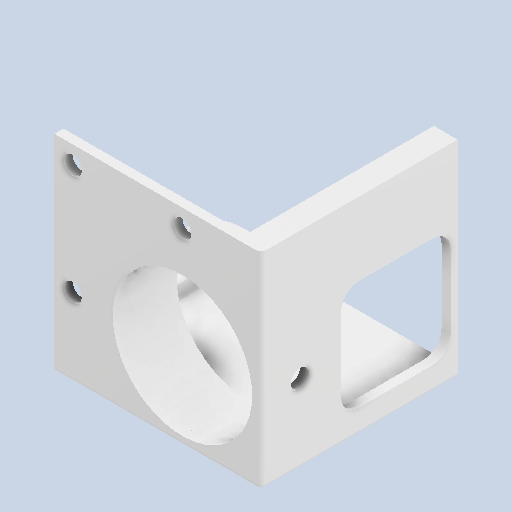
# Autodesk Inventor part: MirrorFix
Saved by Autodesk Inventor 2023 (Build 270158000, 158)
## iProperties
Created: 2022-08-19
Part Number: MirrorFix
Material: ABS Plastic
Document SubType Name: Modeling
Designer: Miner
Density: 1.06 g/cm^3
Appearance: Smooth - White
Author: Miner
Autodesk Inventor part; units mm, degrees
ref_plane "YZ Plane" through (0, 0, 0) normal (1, 0, 0) x (0, 1, 0)
ref_plane "XZ Plane" through (0, 0, 0) normal (0, 1, 0) x (-1, 0, 0)
ref_plane "XY Plane" through (0, 0, 0) normal (0, 0, 1) x (1, 0, 0)
sketch "Sketch1" plane through (0, 0, 0) normal (0, 0, 1) x (1, 0, 0)
  circle A0 centre (0, 0) radius 15 construction
  line L0 (0, 0) -> (0, -12) construction
  line L1 (0, -12) -> (0, 28) construction
  line L2 (0, 28) -> (12, 28) construction
  line L3 (12, 28) -> (-28, 28) construction
  line L4 (-28, 28) -> (-28, -12) construction
  line L5 (-28, -12) -> (12, -12) construction
  line L6 (12, -12) -> (12, 28) construction
  line L7 (-28, 28) -> (17.2, 28)
  line L8 (17.2, 28) -> (17.2, -17.2)
  line L9 (17.2, -17.2) -> (-28, -17.2)
  line L10 (-28, -17.2) -> (-28, 28)
  circle A1 centre (0, 0) radius 15.25
  line L11 (0, -15.25) -> (0, -17.25) construction
  line L12 (-28, -17.2) -> (17.2, -17.2)
  line L13 (17.2, -17.2) -> (17.2, -15.3)
  line L14 (-28, -15.3) -> (-28, -17.2)
  line L15 (17.2, 28) -> (15.3, 28)
  line L16 (17.2, -15.3) -> (17.2, 28)
  circle A2 centre (0, 0) radius 16.85
  line L17 (15.25, 0) -> (17.25, 0) construction
  line L18 (-28, -17.2) -> (17.2, -17.2)
  line L19 (17.2, -17.2) -> (17.2, -15.2)
  line L20 (17.2, -15.2) -> (-28, -15.2)
  line L21 (-28, -15.2) -> (-28, -17.2)
  line L22 (17.2, -15.2) -> (15.2, -15.2)
  line L23 (15.2, -15.2) -> (15.2, 28)
  line L24 (15.2, 28) -> (17.2, 28)
  line L25 (17.2, 28) -> (17.2, -15.2)
  line L26 (-28, -12) -> (-26, -12)
  line L27 (-26, -12) -> (-26, -15.2)
  line L28 (-26, -15.2) -> (-28, -15.2)
  line L29 (-28, -15.2) -> (-28, -12)
  line L30 (15.2, 28) -> (12, 28)
  line L31 (12, 28) -> (12, 26)
  line L32 (12, 26) -> (15.2, 26)
  line L33 (15.2, 26) -> (15.2, 28)
  point P0 (15.2, -7.272)
  point P1 (15.2, 1.2339)
  point P2 (-1.2339, -15.2)
  point P3 (7.272, -15.2)
  point P4 (15.2, 7.272)
  point P5 (-7.272, -15.2)
  point P6 (15.2, -1.2339)
  point P7 (1.2339, -15.2)
  dimension "d0" = 30
  dimension "d1" = 12
  dimension "d2" = 40
  dimension "d3" = 12
  dimension "d4" = 40
  dimension "d5" = 40
  dimension "d6" = 45.2
  dimension "d7" = 45.2
  dimension "d8" = 30.5
  dimension "d22" = 2
  dimension "d30" = 1.6
  dimension "d33" = 2
  dimension "d34" = 2
  dimension "d35" = 2
  dimension "d43" = 2
  dimension "d44" = 2
  constraints: 68 end point, 13 parallel, 9 horizontal, 8 perpendicular, 5 point on line, 3 centre point, 3 vertical, 2 coincident, 2 point on circle
  measures "d0" diameter of A0
  measures "d1" distance of L0.start L0.end
  measures "d2" distance of L0.end L1.end
  measures "d3" distance of L1.end L2.end
  measures "d4" distance of L5.end L4.end
  measures "d5" distance of L4.end L3.end
  measures "d6" distance of L8.end L9.end
  measures "d7" distance of L7.end L8.end
  measures "d8" diameter of A1
  measures "d22" distance of L11.start L11.end
  measures "d30" radial gap between concentric circles of A1 A2
  measures "d33" distance of L17.start L17.end
  measures "d34" distance of L19.end L18.end
  measures "d35" distance of L23.end L24.end
  measures "d43" distance of L27.end L28.end
  measures "d44" distance of L31.end L30.end
extrude "Extrusion1" add sketch "Sketch1" along normal blind 2 contours L7 L31 L32 L23 A2 L20 L27 L26 L10 | L7 L23 L32 L31 | L26 L27 L20 L10 | L7 L8 L20 L23 A2 | L20 A2 L8 L9 L10 | L23 A1 L20 A2 | A2 L23 A1 | L20 A1 A2 | L20 A1 L23 A2 | A2 L23 L20
sketch "Sketch2" plane through (0, 0, 2) normal (0, 0, 1) x (1, 0, 0)
  line L0 (17.2, 28) -> (-28, 28) construction
  line L1 (-28, 28) -> (-28, 24) construction
  line L2 (-28, 28) -> (-28, -17.2) construction
  line L3 (-28, 24) -> (-24, 24) construction
  line L4 (-24, 24) -> (0, 24) construction
  line L5 (-24, 24) -> (-24, 0) construction
  point P0 (0, 0)
  dimension "d11" = 4
  dimension "d12" = 4
  dimension "d13" = 24
  dimension "d14" = 24
  constraints: 8 end point, 3 coincident, 2 point on line, 1 perpendicular, 1 vertical
  measures "d11" distance of L0.end L1.end
  measures "d12" distance of L1.end L3.end
  measures "d13" distance of L3.end L4.end
  measures "d14" distance of L5.start L5.end
hole "Hole1" at (0, 24, 2) at (-24, 24, 2) at (-24, 0, 2) direction (0, 0, -1) diameter 4 end through all
extrude "Extrusion5" add sketch "Sketch1" against normal blind 41 contours L7 L8 L20 L23 A2 | L20 A2 L8 L9 L10 | A2 L23 A1 | L20 A1 A2 | A1 L23 | L20 A1
fillet "Fillet1" radius 1 3 edges at (-5.4, -17.2, 2) (17.2, 5.4, 2) (17.2, -17.2, -19.5)
extrude "Extrusion8" add sketch "Sketch1" against normal blind 41 contours L7 L23 L32 L31 | L26 L27 L20 L10
extrude "Extrusion12" add sketch "Sketch1" against normal blind 12 contours L23 A1 L20 A2 | L20 A1 L23 A2
sketch "Sketch5" plane through (17.2, -16.2, -41) normal (1, 0, 0) x (0, 0, -1)
  line L0 (0, 44.2) -> (0, 0) construction
  line L1 (0, 44.2) -> (0, 16.2) construction
  line L2 (0, 16.2) -> (-13.5, 16.2) construction
  line L3 (-41, 44.2) -> (-41, 42.2) construction
  line L4 (-41, 44.2) -> (-41, 16.2) construction
  line L5 (-41, 16.2) -> (-34.5, 16.2) construction
  circle A0 centre (-34.5, 16.2) radius 2
  line L6 (-25.5, 4.2) -> (-1.5, 4.2)
  line L7 (-1.5, 4.2) -> (-1.5, 28.2)
  line L8 (-1.5, 28.2) -> (-25.5, 28.2)
  line L9 (-25.5, 28.2) -> (-25.5, 4.2)
  line L10 (-25.5, 4.2) -> (-1.5, 28.2) construction
  line L11 (-1.5, 4.2) -> (-25.5, 28.2) construction
  dimension "d64" = 28
  dimension "d65" = 13.5
  dimension "d66" = 6.5
  dimension "d67" = 4
  constraints: 20 end point, 3 perpendicular, 2 parallel, 1 centre point, 1 coincident, 1 horizontal, 1 point on line, 1 vertical
  measures "d64" distance of L0.start L1.end
  measures "d65" distance of L1.end L2.end
  measures "d66" distance of L4.end L5.end
  measures "d67" diameter of A0
extrude "Extrusion14" cut sketch "Sketch5" against normal blind 3
fillet "Fillet2" radius 4 4 edges at (16.2, 12, -15.5) (16.2, -12, -15.5) (16.2, -12, -39.5) (16.2, 12, -39.5)
body "Solid1"
